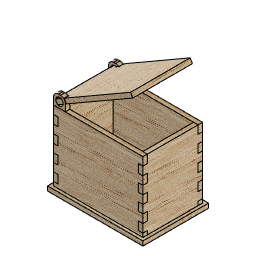
laser cut box with lid v5 (Autodesk Fusion 360 design; units mm, degrees)
Autodesk Fusion 360 part; units mm, degrees
note: some values were not read from the file. Chosen so that the rebuilt part matches the saved one: which face or edge a step refers to; where a step starts. Set by a fixed rule: which sketch regions a step uses.
sketch "base" plane through (0, 0, 0) normal (0, 0, 1) x (1, 0, 0) in component "base"
  line L0 (0, 0) -> (60, 0)
  line L1 (60, 0) -> (60, 40)
  line L2 (60, 40) -> (0, 40)
  line L3 (0, 40) -> (0, 0)
  line L4 (60, 20) -> (0, 20) construction
  line L5 (30, 40) -> (30, 0) construction
  line L6 (-2, 42) -> (62, 42)
  line L7 (62, 42) -> (62, -2)
  line L8 (62, -2) -> (-2, -2)
  line L9 (-2, -2) -> (-2, 42)
  line L10 (-2, 42) -> (62, -2) construction
  line L11 (62, 42) -> (-2, -2) construction
  point P0 (30, 20)
  dimension "d14" = 60
  dimension "d15" = 40
  dimension "d16" = 2
  dimension "d17" = 2
  constraint horizontal L0
  constraint vertical L1
  constraint horizontal L2
  constraint vertical L3
  constraint coincident L0.start L3.end
  constraint midpoint L1 L4.start
  constraint midpoint L3 L4.end
  constraint midpoint L2 L5.start
  constraint midpoint L0 L5.end
  constraint horizontal L6
  constraint perpendicular L6 L7
  constraint parallel L6 L8
  constraint parallel L7 L9
  constraint coincident L10 P0
  constraint coincident L11 P0
  constraint midpoint L4 P0
  measures "d14" distance of L1.end L2.end
  measures "d15" distance of L0.end L1.end
  measures "d16" distance of L2 L6
  measures "d17" distance of L1 L7
extrude "Extrude1" add sketch "base" along normal blind 3 contours L0 L1 L2 L3 | L6 L7 L8 L9 makes body 1 in component "base"
sketch "lenghttabcut" plane through (0, 0, 3) normal (0, 0, 1) x (-1, 0, 0) in component "base"
  line L0 (2, 2) -> (-62, 2)
  line L1 (-62, 2) -> (-62, -42)
  line L2 (-62, -42) -> (2, -42)
  line L3 (2, -42) -> (2, 2)
  line L4 (-6.6667, -40) -> (-13.3333, -40)
  line L5 (-13.3333, -40) -> (-13.3333, -37)
  line L6 (-13.3333, -37) -> (-6.6667, -37)
  line L7 (-6.6667, -37) -> (-6.6667, -40)
  line L8 (-60, -40) -> (0, -40)
  line L9 (0, -40) -> (0, 0)
  dimension "d20" = 6.6667
  dimension "d21" = 6.6667
  dimension "d35" = 3
  constraint horizontal L4
  constraint vertical L5
  constraint horizontal L6
  constraint vertical L7
  constraint collinear L4 L8
  measures "d20" distance of L7 L9
  measures "d21" distance of L4.start L4.end
  measures "d35" distance of L4.start L6.end
extrude "Extrude2" cut sketch "lenghttabcut" against normal blind 3 contours L4 L5 L6 L7 L8 bodies 1 in component "base"
pattern_linear "R-Pattern1" count 4 spacing 13.3333 along (1, 0, 0) of "Extrude2" in component "base"
ref_plane "WorkPlane1" through (30, 40, 1.5) normal (0, 1, 0) x (-1, 0, 0) in component "back"
sketch "back" plane through (30, 40, 1.5) normal (0, 1, 0) x (1, 0, 0) in component "back"
  line L0 (-30, 1.5) -> (30, 1.5)
  line L1 (30, 1.5) -> (30, -48.5)
  line L2 (30, -48.5) -> (-30, -48.5)
  line L3 (-30, -48.5) -> (-30, 1.5)
  point P0 (0, 1.5)
  dimension "d29" = 50
  dimension "d30" = 60
  constraint horizontal L0
  constraint vertical L1
  constraint horizontal L2
  constraint vertical L3
  constraint midpoint L0 P0
  measures "d29" distance of L0.start L2.end
  measures "d30" distance of L1.end L2.end
extrude "Extrude1'" add sketch "back" against normal blind 3 separate body makes body 2 in component "back"
sketch "heighttabcut" plane through (60, 0, 0) normal (1, 0, 0) x (0, 1, 0) in component "back"
  line L0 (40, 0) -> (40, 50)
  line L1 (40, 50) -> (37, 50)
  line L2 (37, 50) -> (37, 0)
  line L3 (37, 0) -> (40, 0)
  line L4 (37, 11.1111) -> (40, 11.1111)
  line L5 (40, 11.1111) -> (40, 5.5556)
  line L6 (40, 5.5556) -> (37, 5.5556)
  line L7 (37, 5.5556) -> (37, 11.1111)
  line L8 (42, 0) -> (-2, 0)
  dimension "d33" = 5.5556
  dimension "d34" = 5.5556
  constraint horizontal L4
  constraint vertical L5
  constraint horizontal L6
  constraint vertical L7
  constraint coincident L0 L5.end
  constraint coincident L2 L4.start
  measures "d33" distance of L6 L8
  measures "d34" distance of L4.end L5.end
combine "Combine1" operation cut target body 2 tool bodies 1 keep tools in component "back"
extrude "Extrude2'" cut sketch "heighttabcut" against normal blind 3 contours L0 L2 L4 L5 L6 L7 bodies 2 in component "back"
pattern_linear "R-Pattern1'" count 4 spacing 11.1111 along (0, 0, 1) of "Extrude2'" in component "back"
extrude "Extrude1''" add 1 faces at (27.8889, 40, 28.7778) along direction (0, 1, 0) blind 3 from surface at -40 separate body on bodies 2 makes body 3 in component "front"
combine "Combine1'" operation cut target body 1 tool bodies 3 keep tools in component "base"
sketch "widthtabcut" plane through (0, 0, 3) normal (0, 0, 1) x (-1, 0, 0) in component "base"
  line L0 (-6.6667, 0) -> (-6.6667, -3)
  line L1 (-6.6667, -3) -> (-13.3333, -3)
  line L2 (-13.3333, -3) -> (-13.3333, 0)
  line L3 (-13.3333, 0) -> (-6.6667, 0)
  line L4 (-20, 0) -> (-20, -3)
  line L5 (-20, -3) -> (-26.6667, -3)
  line L6 (-26.6667, -3) -> (-26.6667, 0)
  line L7 (-26.6667, 0) -> (-20, 0)
  line L8 (-33.3333, 0) -> (-33.3333, -3)
  line L9 (-33.3333, -3) -> (-40, -3)
  line L10 (-40, -3) -> (-40, 0)
  line L11 (-40, 0) -> (-33.3333, 0)
  line L12 (-33.3333, -37) -> (-33.3333, -40)
  line L13 (-33.3333, -40) -> (-40, -40)
  line L14 (-40, -40) -> (-40, -37)
  line L15 (-40, -37) -> (-33.3333, -37)
  line L16 (-20, -37) -> (-20, -40)
  line L17 (-20, -40) -> (-26.6667, -40)
  line L18 (-26.6667, -40) -> (-26.6667, -37)
  line L19 (-26.6667, -37) -> (-20, -37)
  line L20 (-6.6667, -37) -> (-6.6667, -40)
  line L21 (-6.6667, -40) -> (-13.3333, -40)
  line L22 (-13.3333, -40) -> (-13.3333, -37)
  line L23 (-13.3333, -37) -> (-6.6667, -37)
  line L24 (2, 2) -> (-62, 2)
  line L25 (-62, 2) -> (-62, -42)
  line L26 (-62, -42) -> (2, -42)
  line L27 (2, -42) -> (2, 2)
  line L28 (-60, -34.2857) -> (-57, -34.2857)
  line L29 (-57, -34.2857) -> (-57, -28.5714)
  line L30 (-57, -28.5714) -> (-60, -28.5714)
  line L31 (-60, -28.5714) -> (-60, -34.2857)
  line L32 (-60, -40) -> (0, -40)
  line L33 (-60, 0) -> (-60, -40)
  line L34 (-46.6667, 0) -> (-46.6667, -3)
  line L35 (-46.6667, -3) -> (-53.3333, -3)
  line L36 (-53.3333, -3) -> (-53.3333, 0)
  line L37 (-53.3333, 0) -> (-46.6667, 0)
  line L38 (-46.6667, -37) -> (-46.6667, -40)
  line L39 (-46.6667, -40) -> (-53.3333, -40)
  line L40 (-53.3333, -40) -> (-53.3333, -37)
  line L41 (-53.3333, -37) -> (-46.6667, -37)
  dimension "d45" = 3
  dimension "d46" = 5.7143
  dimension "d47" = 5.7143
  constraint horizontal L28
  constraint vertical L29
  constraint horizontal L30
  constraint vertical L31
  constraint collinear L31 L33
  measures "d45" distance of L28.start L28.end
  measures "d46" distance of L28 L32
  measures "d47" distance of L28.start L30.end
extrude "Extrude3" cut sketch "widthtabcut" against normal blind 3 contours L28 L29 L30 L31 L33 bodies 1 in component "base"
pattern_linear "R-Pattern2" count 3 spacing 11.4286 along (0, -1, 0) of "Extrude3" in component "base"
sketch "Sketch1" plane through (60, 0, 0) normal (1, 0, 0) x (0, 1, 0) in component "right"
  line L0 (40, 44.4444) -> (40, 50)
  line L1 (40, 50) -> (37, 50)
  line L2 (37, 50) -> (37, 44.4444)
  line L3 (0, 0) -> (40, 0)
  line L4 (40, 0) -> (40, 50)
  line L5 (40, 50) -> (0, 50)
  line L6 (0, 50) -> (0, 0)
  line L7 (37, 44.4444) -> (40, 44.4444)
  constraint perpendicular L3 L4
  constraint parallel L3 L5
  constraint parallel L4 L6
  constraint horizontal L3
  constraint coincident L3.start L6.end
  constraint coincident L0.end L1.start
extrude "Extrude1'''" add sketch "Sketch1" against normal blind 3 separate body makes body 4 in component "right"
combine "Combine1''" operation cut target body 4 tool bodies 2 keep tools in component "right"
combine "Combine2" operation cut target body 4 tool bodies 3 keep tools in component "right"
combine "Combine3" operation cut target body 4 tool bodies 1 keep tools in component "right"
extrude "Extrude1''''" add 9 faces at (57, 9.5238, 2) (57, 19.0476, 15.8148) (57, 20.9524, 2) (57, 32.381, 2) (57, 1, 18.5185) (57, 1, 29.6296) (57, 2, 40.7407) (57, 38, 20.3704) (57, 38, 31.4815) along direction (-1, 0, 0) blind 3 from surface at -5 separate body start surface through (-2, -2, 0) normal (-1, 0, 0) on bodies 4 makes body 5 in component "left"
combine "Combine2'" operation cut target body 2 tool bodies 5 keep tools in component "back"
combine "Combine1'''" operation cut target body 3 tool bodies 5 keep tools in component "front"
combine "Combine2''" operation cut target body 1 tool bodies 5 keep tools in component "base"
sketch "Sketch6" plane through (0, 37, 0) normal (0, -1, 0) x (1, 0, 0) in component "back"
  line L0 (3, 44.4444) -> (3, 38.8889)
  line L1 (3, 38.8889) -> (0, 38.8889)
  line L2 (0, 38.8889) -> (0, 33.3333)
  line L3 (0, 33.3333) -> (3, 33.3333)
  line L4 (3, 33.3333) -> (3, 27.7778)
  line L5 (3, 27.7778) -> (0, 27.7778)
  line L6 (0, 27.7778) -> (0, 22.2222)
  line L7 (0, 22.2222) -> (3, 22.2222)
  line L8 (3, 22.2222) -> (3, 16.6667)
  line L9 (3, 16.6667) -> (0, 16.6667)
  line L10 (0, 16.6667) -> (0, 11.1111)
  line L11 (0, 11.1111) -> (3, 11.1111)
  line L12 (3, 11.1111) -> (3, 5.5556)
  line L13 (3, 5.5556) -> (0, 5.5556)
  line L14 (0, 5.5556) -> (0, 3)
  line L15 (0, 3) -> (6.6667, 3)
  line L16 (6.6667, 3) -> (6.6667, 0)
  line L17 (6.6667, 0) -> (13.3333, 0)
  line L18 (13.3333, 0) -> (13.3333, 3)
  line L19 (13.3333, 3) -> (20, 3)
  line L20 (20, 3) -> (20, 0)
  line L21 (20, 0) -> (26.6667, 0)
  line L22 (26.6667, 0) -> (26.6667, 3)
  line L23 (26.6667, 3) -> (33.3333, 3)
  line L24 (33.3333, 3) -> (33.3333, 0)
  line L25 (33.3333, 0) -> (40, 0)
  line L26 (40, 0) -> (40, 3)
  line L27 (40, 3) -> (46.6667, 3)
  line L28 (46.6667, 3) -> (46.6667, 0)
  line L29 (46.6667, 0) -> (53.3333, 0)
  line L30 (53.3333, 0) -> (53.3333, 3)
  line L31 (53.3333, 3) -> (60, 3)
  line L32 (60, 3) -> (60, 5.5556)
  line L33 (60, 5.5556) -> (57, 5.5556)
  line L34 (57, 5.5556) -> (57, 11.1111)
  line L35 (57, 11.1111) -> (60, 11.1111)
  line L36 (60, 11.1111) -> (60, 16.6667)
  line L37 (60, 16.6667) -> (57, 16.6667)
  line L38 (57, 16.6667) -> (57, 22.2222)
  line L39 (57, 22.2222) -> (60, 22.2222)
  line L40 (60, 22.2222) -> (60, 27.7778)
  line L41 (60, 27.7778) -> (57, 27.7778)
  line L42 (57, 27.7778) -> (57, 33.3333)
  line L43 (57, 33.3333) -> (60, 33.3333)
  line L44 (60, 33.3333) -> (60, 38.8889)
  line L45 (60, 38.8889) -> (57, 38.8889)
  line L46 (57, 38.8889) -> (57, 44.4444)
  line L47 (57, 44.4444) -> (60, 44.4444)
  line L48 (60, 44.4444) -> (60, 50)
  line L49 (60, 50) -> (0, 50)
  line L50 (0, 50) -> (0, 44.4444)
  line L51 (0, 44.4444) -> (3, 44.4444)
  line L52 (8, 50) -> (0, 50)
  line L53 (0, 50) -> (0, 58)
  line L54 (0, 58) -> (8, 58)
  line L55 (8, 58) -> (8, 50)
  line L56 (8, 50) -> (0, 58) construction
  line L57 (0, 50) -> (8, 58) construction
  circle A0 centre (4, 54) radius 2.5
  point P0 (4, 54)
  dimension "d75" = 5
  dimension "d76" = 4
  dimension "d77" = 4
  constraint horizontal L52
  constraint perpendicular L52 L53
  constraint parallel L52 L54
  constraint parallel L53 L55
  constraint coincident L56 P0
  constraint coincident L57 P0
  constraint coincident P0 A0.centre
  constraint collinear L49 L52
  constraint coincident L49.end L50.start
  measures "d75" diameter of A0
  measures "d76" distance of L54 P0
  measures "d77" distance of L55 P0
extrude "Extrude4" add sketch "Sketch6" against normal blind 3 separate body contours L49 L52 L53 L54 L55 makes body 6 in component "back"
fillet "Fillet1" radius 3.3333 2 edges at (8, 38.5, 58) (0, 38.5, 58) on bodies 6 in component "back"
extrude "Extrude3'" add 1 faces at (4.0623, 37, 50.5023) along direction (0, -1, 0) blind 3 from surface at 34 separate body on bodies 6 makes body 7 in component "front"
ref_plane "WorkPlane1" through (30, 1.5, 54) normal (0, 0, 1) x (1, 0, 0) in component "lid"
sketch "Sketch1 (2)" plane through (30, 1.5, 54) normal (0, 0, 1) x (1, 0, 0) in component "lid"
  line L0 (-28.5, 38.5) -> (30, 38.5)
  line L1 (30, 38.5) -> (30, -1.5)
  line L2 (30, -1.5) -> (-28.5, -1.5)
  line L3 (-28.5, -1.5) -> (-28.5, 38.5)
  line L4 (30, 35.5) -> (30, 1.5)
  line L5 (30, 38.5) -> (-30, 38.5)
  line L6 (-30, -1.5) -> (30, -1.5)
  line L7 (-23.5, -1.5) -> (-28.5, -1.5)
  line L8 (-28.5, 1.5) -> (-23.5, 1.5)
  line L9 (-23.5, -1.5) -> (-23.6741, 38.5) construction
  line L10 (-23.5, -1.5) -> (-21.5, -1.5)
  line L11 (-21.5, -1.5) -> (-21.5, 1.5)
  line L12 (-21.5, 1.5) -> (-23.5, 1.5)
  line L13 (-23.5, 1.5) -> (-23.5, -1.5)
  line L14 (30, 18.5) -> (-28.5, 18.5) construction
  line L15 (-21.5, 35.5) -> (-23.5, 35.5)
  line L16 (-21.5, 38.5) -> (-21.5, 35.5)
  line L17 (-23.5, 38.5) -> (-21.5, 38.5)
  line L18 (-23.5, 35.5) -> (-23.5, 38.5)
  dimension "d85" = 3
  dimension "d86" = 2
  constraint horizontal L0
  constraint vertical L1
  constraint horizontal L2
  constraint vertical L3
  constraint collinear L1 L4
  constraint collinear L0 L5
  constraint collinear L2 L6
  constraint coincident L3 L2.end
  constraint coincident L7.start L9.start
  constraint coincident L0 L9.end
  constraint horizontal L10
  constraint vertical L11
  constraint horizontal L12
  constraint vertical L13
  constraint midpoint L1 L14.start
  constraint midpoint L3 L14.end
  constraint symmetric L7.start L14 L17.start
  constraint symmetric L10.end L14 L16.start
  constraint symmetric L11.end L14 L15.start
  constraint symmetric L8.end L14 L15.end
  measures "d85" distance of L10.end L11.end
  measures "d86" distance of L11.end L8.end
extrude "Extrude1'''''" add sketch "Sketch1 (2)" along normal mid plane 3 separate body contours L0 L1 L2 L3 L4 L5 L6 L8 L11 L12 L15 L16 L18 | L2 L3 L6 L7 L8 L13 makes body 8 in component "lid"
combine "Combine1''''" operation cut target body 8 tool bodies 6 keep tools in component "lid"
combine "Combine2'''" operation cut target body 8 tool bodies 7 keep tools in component "lid"
move_body "Move1" bodies 8 to x (0.866025, 0, 0.5) y (0, 1, 0) z (-0.5, 0, 0.866025) at (27.5359, 0, 5.2346) in component "lid"
sketch "Sketch4" plane through (0, 40, 0) normal (0, 1, 0) x (-1, 0, 0) in component "back"
  line L0 (-3, 44.4444) -> (0, 44.4444)
  line L1 (0, 44.4444) -> (0, 50)
  line L2 (0, 50) -> (-60, 50)
  line L3 (-60, 50) -> (-60, 44.4444)
  line L4 (-60, 44.4444) -> (-57, 44.4444)
  line L5 (-57, 44.4444) -> (-57, 38.8889)
  line L6 (-57, 38.8889) -> (-60, 38.8889)
  line L7 (-60, 38.8889) -> (-60, 33.3333)
  line L8 (-60, 33.3333) -> (-57, 33.3333)
  line L9 (-57, 33.3333) -> (-57, 27.7778)
  line L10 (-57, 27.7778) -> (-60, 27.7778)
  line L11 (-60, 27.7778) -> (-60, 22.2222)
  line L12 (-60, 22.2222) -> (-57, 22.2222)
  line L13 (-57, 22.2222) -> (-57, 16.6667)
  line L14 (-57, 16.6667) -> (-60, 16.6667)
  line L15 (-60, 16.6667) -> (-60, 11.1111)
  line L16 (-60, 11.1111) -> (-57, 11.1111)
  line L17 (-57, 11.1111) -> (-57, 5.5556)
  line L18 (-57, 5.5556) -> (-60, 5.5556)
  line L19 (-60, 5.5556) -> (-60, 3)
  line L20 (-60, 3) -> (-53.3333, 3)
  line L21 (-53.3333, 3) -> (-53.3333, 0)
  line L22 (-53.3333, 0) -> (-46.6667, 0)
  line L23 (-46.6667, 0) -> (-46.6667, 3)
  line L24 (-46.6667, 3) -> (-40, 3)
  line L25 (-40, 3) -> (-40, 0)
  line L26 (-40, 0) -> (-33.3333, 0)
  line L27 (-33.3333, 0) -> (-33.3333, 3)
  line L28 (-33.3333, 3) -> (-26.6667, 3)
  line L29 (-26.6667, 3) -> (-26.6667, 0)
  line L30 (-26.6667, 0) -> (-20, 0)
  line L31 (-20, 0) -> (-20, 3)
  line L32 (-20, 3) -> (-13.3333, 3)
  line L33 (-13.3333, 3) -> (-13.3333, 0)
  line L34 (-13.3333, 0) -> (-6.6667, 0)
  line L35 (-6.6667, 0) -> (-6.6667, 3)
  line L36 (-6.6667, 3) -> (0, 3)
  line L37 (0, 3) -> (0, 5.5556)
  line L38 (0, 5.5556) -> (-3, 5.5556)
  line L39 (-3, 5.5556) -> (-3, 11.1111)
  line L40 (-3, 11.1111) -> (0, 11.1111)
  line L41 (0, 11.1111) -> (0, 16.6667)
  line L42 (0, 16.6667) -> (-3, 16.6667)
  line L43 (-3, 16.6667) -> (-3, 22.2222)
  line L44 (-3, 22.2222) -> (0, 22.2222)
  line L45 (0, 22.2222) -> (0, 27.7778)
  line L46 (0, 27.7778) -> (-3, 27.7778)
  line L47 (-3, 27.7778) -> (-3, 33.3333)
  line L48 (-3, 33.3333) -> (0, 33.3333)
  line L49 (0, 33.3333) -> (0, 38.8889)
  line L50 (0, 38.8889) -> (-3, 38.8889)
  line L51 (-3, 38.8889) -> (-3, 44.4444)
sketch "Sketch5" plane through (0, 40, 0) normal (0, 1, 0) x (-1, 0, 0) in component "back"
  line L0 (-3, 44.4444) -> (0, 44.4444)
  line L1 (0, 44.4444) -> (0, 50)
  line L2 (0, 50) -> (-60, 50)
  line L3 (-60, 50) -> (-60, 44.4444)
  line L4 (-60, 44.4444) -> (-57, 44.4444)
  line L5 (-57, 44.4444) -> (-57, 38.8889)
  line L6 (-57, 38.8889) -> (-60, 38.8889)
  line L7 (-60, 38.8889) -> (-60, 33.3333)
  line L8 (-60, 33.3333) -> (-57, 33.3333)
  line L9 (-57, 33.3333) -> (-57, 27.7778)
  line L10 (-57, 27.7778) -> (-60, 27.7778)
  line L11 (-60, 27.7778) -> (-60, 22.2222)
  line L12 (-60, 22.2222) -> (-57, 22.2222)
  line L13 (-57, 22.2222) -> (-57, 16.6667)
  line L14 (-57, 16.6667) -> (-60, 16.6667)
  line L15 (-60, 16.6667) -> (-60, 11.1111)
  line L16 (-60, 11.1111) -> (-57, 11.1111)
  line L17 (-57, 11.1111) -> (-57, 5.5556)
  line L18 (-57, 5.5556) -> (-60, 5.5556)
  line L19 (-60, 5.5556) -> (-60, 3)
  line L20 (-60, 3) -> (-53.3333, 3)
  line L21 (-53.3333, 3) -> (-53.3333, 0)
  line L22 (-53.3333, 0) -> (-46.6667, 0)
  line L23 (-46.6667, 0) -> (-46.6667, 3)
  line L24 (-46.6667, 3) -> (-40, 3)
  line L25 (-40, 3) -> (-40, 0)
  line L26 (-40, 0) -> (-33.3333, 0)
  line L27 (-33.3333, 0) -> (-33.3333, 3)
  line L28 (-33.3333, 3) -> (-26.6667, 3)
  line L29 (-26.6667, 3) -> (-26.6667, 0)
  line L30 (-26.6667, 0) -> (-20, 0)
  line L31 (-20, 0) -> (-20, 3)
  line L32 (-20, 3) -> (-13.3333, 3)
  line L33 (-13.3333, 3) -> (-13.3333, 0)
  line L34 (-13.3333, 0) -> (-6.6667, 0)
  line L35 (-6.6667, 0) -> (-6.6667, 3)
  line L36 (-6.6667, 3) -> (0, 3)
  line L37 (0, 3) -> (0, 5.5556)
  line L38 (0, 5.5556) -> (-3, 5.5556)
  line L39 (-3, 5.5556) -> (-3, 11.1111)
  line L40 (-3, 11.1111) -> (0, 11.1111)
  line L41 (0, 11.1111) -> (0, 16.6667)
  line L42 (0, 16.6667) -> (-3, 16.6667)
  line L43 (-3, 16.6667) -> (-3, 22.2222)
  line L44 (-3, 22.2222) -> (0, 22.2222)
  line L45 (0, 22.2222) -> (0, 27.7778)
  line L46 (0, 27.7778) -> (-3, 27.7778)
  line L47 (-3, 27.7778) -> (-3, 33.3333)
  line L48 (-3, 33.3333) -> (0, 33.3333)
  line L49 (0, 33.3333) -> (0, 38.8889)
  line L50 (0, 38.8889) -> (-3, 38.8889)
  line L51 (-3, 38.8889) -> (-3, 44.4444)
  circle A0 centre (-7, 46) radius 2.5
  dimension "d64" = 5
  dimension "d65" = 4
  dimension "d66" = 4
  measures "d64" diameter of A0
  measures "d65" distance of L51 A0.centre
  measures "d66" distance of L2 A0.centre
extrude "Extrude3''" [rolled back] along distance -46 taper angle 0 in component "back"
combine "Combine4" [rolled back] in component "right"
component "base" placed x (1, 0, 0) y (0, 1, 0) z (0, 0, 1) at (0, 0, 0)
component "back" placed x (1, 0, 0) y (0, 1, 0) z (0, 0, 1) at (0, 0, 0)
component "front" placed x (1, 0, 0) y (0, 1, 0) z (0, 0, 1) at (0, 0, 0)
component "right" placed x (1, 0, 0) y (0, 1, 0) z (0, 0, 1) at (0, 0, 0)
component "left" placed x (1, 0, 0) y (0, 1, 0) z (0, 0, 1) at (0, 0, 0)
component "lid" placed x (1, 0, 0) y (0, 1, 0) z (0, 0, 1) at (0, 0, 0)
equation "length = 60 mm" comment "exterior"
equation "width = 40 mm" comment "exterior"
equation "height = 50 mm" comment "exterior"
equation "thick = 3 mm" comment "material thickness"
equation "Ltab = 4" comment "No. tab"
equation "Wtab = 3" comment "No. tab"
equation "Htab = 4" comment "No. tab"
equation "WtabWidth = width / ( ( Wtab * 2 ) + 1 )" comment "tab size"
equation "LtabWidth = length / ( ( Ltab * 2 ) + 1 )" comment "tab size"
equation "HtabWidth = height / ( ( Htab * 2 ) + 1 )" comment "tab size"
equation "baseoffset = 2 mm" comment "Base outline"
equation "d14 = length"
equation "d15 = width"
equation "d16 = baseoffset"
equation "d17 = baseoffset"
equation "d18 = thick"
equation "d20 = LtabWidth"
equation "d21 = LtabWidth"
equation "d22 = -thick"
equation "d24 = Ltab"
equation "d26 = length - LtabWidth * 3"
equation "d28 = -baseoffset"
equation "d29 = height"
equation "d30 = length"
equation "d31 = -thick"
equation "d33 = HtabWidth"
equation "d34 = HtabWidth"
equation "d35 = thick"
equation "d36 = -thick"
equation "d38 = Htab"
equation "d40 = height - HtabWidth * 3"
equation "d42 = -baseoffset"
equation "d43 = thick"
equation "d45 = thick"
equation "d46 = WtabWidth"
equation "d47 = WtabWidth"
equation "d48 = -thick"
equation "d50 = Wtab"
equation "d52 = width - WtabWidth * 3"
equation "d54 = -thick"
equation "d56 = -baseoffset - thick"
equation "d57 = thick"
equation "Hingedia = 5 mm"
equation "Hineoffset = Hingedia / 2 + thick / 2"
equation "d64 = Hingedia"
equation "d65 = Hineoffset"
equation "d66 = Hineoffset"
equation "d67 = -( thick * 2 + width )"
equation "d69 = -( thick * 2 + width )"
equation "d75 = Hingedia"
equation "d76 = Hineoffset"
equation "d77 = Hineoffset"
equation "d78 = -thick"
equation "d81 = Hingedia / 1.5"
equation "d82 = -thick"
equation "d83 = thick"
equation "d85 = thick"
equation "d86 = Hineoffset / 2"
equation "d87 = thick"
